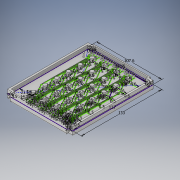
# Autodesk Inventor part: 24WellOneLayerFluidics5x4V2
Saved by Autodesk Inventor 2018 (Build 220112000, 112)
## iProperties
Created: 2019-12-20
Part Number: 24WellOneLayerFluidics5x4V2
Material: Generic
Document SubType Name: Modeling
Designer: Sergio
Density: 1 g/cm^3
Appearance: Default
Author: Sergio
Autodesk Inventor part; units mm, degrees
(part 1 of 4)
ref_plane "YZ Plane" through (0, 0, 0) normal (1, 0, 0) x (0, 1, 0)
ref_plane "XZ Plane" through (0, 0, 0) normal (0, 1, 0) x (-1, 0, 0)
ref_plane "XY Plane" through (0, 0, 0) normal (0, 0, 1) x (1, 0, 0)
sketch "Sketch2" plane through (0, 0, 0) normal (0, 1, 0) x (-1, 0, 0)
  line L0 (-50.8, 63.5) -> (-50.8, -63.5) construction
  line L1 (-50.8, -63.5) -> (50.8, -63.5) construction
  line L2 (50.8, -63.5) -> (50.8, 63.5) construction
  line L3 (50.8, 63.5) -> (-50.8, 63.5) construction
  line L4 (-50.8, 63.5) -> (50.8, -63.5) construction
  line L5 (-50.8, -63.5) -> (50.8, 63.5) construction
  line L6 (-53.8, 66.5) -> (-53.8, -66.5) construction
  line L7 (-53.8, -66.5) -> (53.8, -66.5) construction
  line L8 (53.8, -66.5) -> (53.8, 66.5) construction
  line L9 (53.8, 66.5) -> (-53.8, 66.5) construction
  line L10 (-53.8, 66.5) -> (53.8, -66.5) construction
  line L11 (-53.8, -66.5) -> (53.8, 66.5) construction
  line L12 (53.8, 66.5) -> (46.8, 66.5) construction
  line L13 (50.8, 63.5) -> (44.8, 63.5) construction
  line L14 (44.8, 63.5) -> (44.8, 67) construction
  line L15 (46.8, 66.5) -> (46.8, 69) construction
  line L16 (-53.8, 66.5) -> (-46.8, 66.5) construction
  line L17 (-50.8, 63.5) -> (-44.8, 63.5) construction
  line L18 (-46.8, 66.5) -> (-46.8, 69) construction
  line L19 (-44.8, 63.5) -> (-44.8, 67) construction
  line L20 (-53.8, -66.5) -> (-46.8, -66.5) construction
  line L21 (-50.8, -63.5) -> (-44.8, -63.5) construction
  line L22 (-46.8, -66.5) -> (-46.8, -69) construction
  line L23 (-44.8, -63.5) -> (-44.8, -67) construction
  line L24 (53.8, -66.5) -> (46.8, -66.5) construction
  line L25 (50.8, -63.5) -> (44.8, -63.5) construction
  line L26 (46.8, -66.5) -> (46.8, -69) construction
  line L27 (44.8, -63.5) -> (44.8, -67) construction
  line L28 (46.8, 69) -> (-46.8, 69) construction
  line L29 (-44.8, 67) -> (44.8, 67) construction
  line L30 (44.8, -67) -> (-44.8, -67) construction
  line L31 (-46.8, -69) -> (46.8, -69) construction
  point P0 (0, 0)
  dimension "d21" = 127
  dimension "d22" = 101.6
  dimension "d23" = 133
  dimension "d24" = 107.6
  dimension "d25" = 7
  dimension "d26" = 6
  dimension "d27" = 3.5
  dimension "d28" = 2.5
  dimension "d29" = 7
  dimension "d30" = 6
  dimension "d31" = 2.5
  dimension "d32" = 3.5
  dimension "d33" = 7
  dimension "d34" = 6
  dimension "d35" = 2.5
  dimension "d36" = 3.5
  dimension "d37" = 7
  dimension "d38" = 6
  dimension "d39" = 2.5
  dimension "d40" = 3.5
  constraints: 64 end point, 9 vertical, 8 point on line, 4 midpoint, 4 parallel, 3 perpendicular
  measures "d21" distance of L0.start L0.end
  measures "d22" distance of L1.end L0.end
  measures "d23" distance of L6.start L6.end
  measures "d24" distance of L7.end L6.end
  measures "d25" distance of L8.end L12.end
  measures "d26" distance of L2.end L13.end
  measures "d27" distance of L13.end L14.end
  measures "d28" distance of L12.end L15.end
  measures "d29" distance of L6.start L16.end
  measures "d30" distance of L0.start L17.end
  measures "d31" distance of L16.end L18.end
  measures "d32" distance of L17.end L19.end
  measures "d33" distance of L6.end L20.end
  measures "d34" distance of L0.end L21.end
  measures "d35" distance of L20.end L22.end
  measures "d36" distance of L21.end L23.end
  measures "d37" distance of L7.end L24.end
  measures "d38" distance of L1.end L25.end
  measures "d39" distance of L24.end L26.end
  measures "d40" distance of L25.end L27.end
sketch "Sketch3" plane through (0, 0, 0) normal (0, 1, 0) x (-1, 0, 0)
  line L0 (50.8, 63.5) -> (-50.8, 63.5) construction
  line L1 (-50.8, -63.5) -> (50.8, -63.5) construction
  line L2 (50.8, -63.5) -> (50.8, 63.5) construction
  line L3 (-53.8, 66.5) -> (-53.8, -66.5) construction
  line L4 (53.8, -66.5) -> (53.8, 66.5) construction
  line L5 (53.8, 66.5) -> (-53.8, 66.5) construction
  line L6 (-44.8, 67) -> (44.8, 67) construction
  line L7 (46.8, 69) -> (-46.8, 69) construction
  line L8 (-46.8, -69) -> (46.8, -69) construction
  line L9 (44.8, -67) -> (-44.8, -67) construction
  line L10 (46.8, 69) -> (-46.8, 69)
  line L11 (46.8, -69) -> (-46.8, -69)
  line L12 (46.8, 66.5) -> (46.8, 69) construction
  line L13 (44.8, 63.5) -> (44.8, 67) construction
  line L14 (50.8, 63.5) -> (44.8, 63.5) construction
  line L15 (53.8, 66.5) -> (46.8, 66.5) construction
  line L16 (46.8, 69) -> (46.8, 66.5)
  line L17 (46.8, 66.5) -> (53.8, 66.5)
  line L18 (53.8, 66.5) -> (53.8, -66.5)
  line L19 (53.8, -66.5) -> (46.8, -66.5)
  line L20 (46.8, -66.5) -> (46.8, -69)
  line L21 (-46.8, -69) -> (-46.8, -66.5)
  line L22 (-46.8, -66.5) -> (-53.8, -66.5)
  line L23 (-53.8, 66.5) -> (-53.8, -66.5)
  line L24 (-46.8, 69) -> (-46.8, 66.5)
  line L25 (-53.8, 66.5) -> (-46.8, 66.5)
  line L26 (-44.8, 67) -> (-44.8, 63.5)
  line L27 (-44.8, 63.5) -> (-50.8, 63.5)
  line L28 (-50.8, 63.5) -> (-50.8, -63.5) construction
  line L29 (-44.8, -63.5) -> (-44.8, -67) construction
  line L30 (-44.8, -63.5) -> (-44.8, -67)
  line L31 (-44.8, -63.5) -> (-50.8, -63.5)
  line L32 (-50.8, -63.5) -> (-50.8, 63.5)
  line L33 (-44.8, 67) -> (44.8, 67)
  line L34 (44.8, 67) -> (44.8, 63.5)
  line L35 (44.8, 63.5) -> (50.8, 63.5)
  line L36 (50.8, 63.5) -> (50.8, -63.5)
  line L37 (50.8, -63.5) -> (44.8, -63.5)
  line L38 (44.8, -63.5) -> (44.8, -67)
  line L39 (44.8, -67) -> (-44.8, -67)
  line L40 (44.8, 63.5) -> (-44.8, 63.5)
  line L41 (44.8, -63.5) -> (-44.8, -63.5)
  line L42 (-44.8, -63.5) -> (44.8, -63.5)
  line L43 (44.8, -63.5) -> (44.8, -64.25)
  line L44 (44.8, -64.25) -> (-44.8, -64.25)
  line L45 (-44.8, -64.25) -> (-44.8, -63.5)
  point P0 (0, 0)
  dimension "d547" = 89.6
  dimension "d548" = 0.75
  constraints: 60 end point, 11 perpendicular, 9 collinear, 7 point on line, 5 parallel, 2 horizontal, 1 vertical
  measures "d547" distance of L43.end L44.end
  measures "d548" distance of L42.end L43.end
extrude "Extrusion1" add sketch "Sketch3" along normal blind 6 and the other way blind 8
extrude "Extrusion2" add sketch "Sketch3" against normal blind 8 contours L33 L34 L40 L26 | L40 L35 L36 L37 L41 L31 L32 L27 | L41 L38 L44 L30 | L44 L38 L39 L30
sketch "Sketch5" plane through (0, 0, 0) normal (0, 1, 0) x (1, 0, 0)
  line L0 (-50.8, 63.5) -> (-44.8, 63.5) construction
  line L1 (-50.8, 63.5) -> (-41.305, 63.5) construction
  line L2 (-50.8, 60.019) -> (-50.8, 63.5) construction
  line L3 (-50.8, -63.5) -> (-50.8, 63.5) construction
  line L4 (-50.8, -63.5) -> (-29.25, -63.5) construction
  line L5 (-29.25, -63.5) -> (-29.25, -48.75) construction
  line L6 (-29.25, -48.75) -> (-50.8, -48.75) construction
  line L7 (-50.8, -48.75) -> (-50.8, -63.5) construction
  circle A0 centre (-29.25, -48.75) radius 2.8 construction
  line L8 (-29.25, -48.75) -> (-29.25, -29.25) construction
  circle A1 centre (-29.25, -29.25) radius 2.8 construction
  line L9 (-29.25, -29.25) -> (-29.25, -9.75) construction
  line L10 (-29.25, -9.75) -> (-29.25, 9.75) construction
  line L11 (-29.25, 9.75) -> (-29.25, 29.25) construction
  line L12 (-29.25, 29.25) -> (-29.25, 48.75) construction
  circle A2 centre (-29.25, -9.75) radius 2.8 construction
  circle A3 centre (-29.25, 9.75) radius 2.8 construction
  circle A4 centre (-29.25, 29.25) radius 2.8 construction
  circle A5 centre (-29.25, 48.75) radius 2.8 construction
  line L13 (-29.25, 48.75) -> (-9.75, 48.75) construction
  line L14 (-9.75, 48.75) -> (9.75, 48.75) construction
  line L15 (9.75, 48.75) -> (29.25, 48.75) construction
  circle A6 centre (-9.75, 48.75) radius 2.8 construction
  circle A7 centre (9.75, 48.75) radius 2.8 construction
  circle A8 centre (29.25, 48.75) radius 2.8 construction
  circle A9 centre (-9.75, -48.75) radius 2.8 construction
  circle A10 centre (-9.75, -29.25) radius 2.8 construction
  circle A11 centre (-9.75, -9.75) radius 2.8 construction
  circle A12 centre (-9.75, 9.75) radius 2.8 construction
  circle A13 centre (-9.75, 29.25) radius 2.8 construction
  circle A14 centre (9.75, -48.75) radius 2.8 construction
  circle A15 centre (9.75, -29.25) radius 2.8 construction
  circle A16 centre (9.75, -9.75) radius 2.8 construction
  circle A17 centre (9.75, 9.75) radius 2.8 construction
  circle A18 centre (9.75, 29.25) radius 2.8 construction
  circle A19 centre (29.25, -48.75) radius 2.8 construction
  circle A20 centre (29.25, -29.25) radius 2.8 construction
  circle A21 centre (29.25, -9.75) radius 2.8 construction
  circle A22 centre (29.25, 9.75) radius 2.8 construction
  circle A23 centre (29.25, 29.25) radius 2.8 construction
  circle A24 centre (29.25, 29.25) radius 2.8 construction
  circle A25 centre (29.25, 48.75) radius 2.8 construction
  circle A26 centre (29.25, -29.25) radius 2.8 construction
  circle A27 centre (29.25, -48.75) radius 2.8 construction
  line L16 (26.45, -48.75) -> (25.391, -48.75) construction
  line L17 (-29.2495, -4.9541) -> (-29.2495, -4.4541) construction
  point P0 (0, 0)
  dimension "d49" = 21.55
  dimension "d50" = 14.75
  dimension "d51" = 5.6
  dimension "d52" = 19.5
  dimension "d53" = 5.6
  dimension "d54" = 19.5
  dimension "d55" = 19.5
  dimension "d56" = 19.5
  dimension "d57" = 19.5
  dimension "d58" = 5.6
  dimension "d59" = 5.6
  dimension "d60" = 5.6
  dimension "d61" = 5.6
  dimension "d62" = 19.5
  dimension "d63" = 19.5
  dimension "d64" = 19.5
  dimension "d65" = 5.6
  dimension "d66" = 5.6
  dimension "d67" = 5.6
  dimension "d68" = 5.6
  dimension "d69" = 5.6
  dimension "d70" = 5.6
  dimension "d71" = 5.6
  dimension "d72" = 5.6
  dimension "d73" = 5.6
  dimension "d74" = 5.6
  dimension "d75" = 5.6
  dimension "d76" = 5.6
  dimension "d77" = 5.6
  dimension "d78" = 5.6
  dimension "d79" = 5.6
  dimension "d80" = 5.6
  dimension "d81" = 5.6
  dimension "d82" = 5.6
  dimension "d88" = 1.059
  constraints: 32 end point, 27 centre point, 9 coincident, 5 point on line, 3 horizontal, 2 parallel, 2 vertical, 1 horizontal alignment, 1 perpendicular, 2 other
  measures "d49" distance of L6.end L5.end
  measures "d50" distance of L5.end L4.end
  measures "d51" diameter of A0
  measures "d52" distance of L8.start L8.end
  measures "d53" diameter of A1
  measures "d54" distance of L9.start L9.end
  measures "d55" distance of L9.end L10.end
  measures "d56" distance of L10.end L11.end
  measures "d57" distance of L11.end L12.end
  measures "d58" diameter of A2
  measures "d59" diameter of A3
  measures "d60" diameter of A4
  measures "d61" diameter of A5
  measures "d62" distance of L13.start L13.end
  measures "d63" distance of L13.end L14.end
  measures "d64" distance of L14.end L15.end
  measures "d65" diameter of A6
  measures "d66" diameter of A7
  measures "d67" diameter of A8
  measures "d68" diameter of A9
  measures "d69" diameter of A10
  measures "d70" diameter of A11
  measures "d71" diameter of A12
  measures "d72" diameter of A13
  measures "d73" diameter of A14
  measures "d74" diameter of A15
  measures "d75" diameter of A16
  measures "d76" diameter of A17
  measures "d77" diameter of A18
  measures "d78" diameter of A19
  measures "d79" diameter of A20
  measures "d80" diameter of A21
  measures "d81" diameter of A22
  measures "d82" diameter of A23
  measures "d88" distance of L16.start L16.end
sketch "Sketch6" plane through (0, 0, 0) normal (0, 1, 0) x (1, 0, 0)
  circle A0 centre (35.0419, -55.5191) radius 0.75 construction
  line L0 (35.0419, -55.5191) -> (35.0419, -60.0514) construction
  circle A1 centre (37.3055, -60.0191) radius 0.75 construction
  circle A2 centre (33.3055, -60.0191) radius 0.75 construction
  line L1 (33.3055, -60.0191) -> (37.3055, -60.0191) construction
  circle A3 centre (29.25, 29.25) radius 2.8 construction
  circle A4 centre (29.25, 48.75) radius 2.8 construction
  circle A5 centre (29.25, -29.25) radius 2.8 construction
  circle A6 centre (29.25, -48.75) radius 2.8 construction
  circle A7 centre (29.3055, -60.0191) radius 0.75 construction
  line L2 (34.4097, -49.3098) -> (34.4156, -25.002) construction
  line L3 (35.7822, -49.2776) -> (35.7822, -7.8641) construction
  line L4 (37.0912, 9.3686) -> (37.0912, -49.2776) construction
  line L5 (38.4002, 26.6014) -> (38.4002, -49.2776) construction
  line L6 (26.45, -48.75) -> (25.391, -48.75) construction
  line L7 (33.3055, -60.0191) -> (37.3055, -60.0191) construction
  line L8 (35.0419, -55.5191) -> (39.0419, -55.5191) construction
  line L9 (37.3055, -60.0191) -> (41.3055, -60.0191) construction
  circle A8 centre (41.3055, -60.0191) radius 0.75 construction
  line L10 (29.25, -35.55) -> (33.1642, -42.2012) construction
  line L11 (34.4097, -49.3098) -> (35.0419, -50.4326) construction
  line L12 (35.0419, -55.5191) -> (35.0419, -50.4326) construction
  line L13 (29.25, -16.05) -> (34.4156, -25.002) construction
  line L14 (37.3055, -60.0191) -> (37.3055, -51.916) construction
  line L15 (29.25, 3.45) -> (35.7822, -7.8641) construction
  line L16 (29.25, 22.95) -> (37.0912, 9.3686) construction
  line L17 (29.25, 42.45) -> (38.4002, 26.6014) construction
  line L18 (39.0419, -55.5191) -> (39.0419, -52.6564) construction
  line L19 (39.0419, -52.6564) -> (37.0912, -49.2776) construction
  line L20 (41.3055, -60.0191) -> (41.3055, -54.3097) construction
  line L21 (38.4002, -49.2776) -> (41.3055, -54.3097) construction
  line L22 (35.7822, -49.2776) -> (37.3055, -51.916) construction
  line L23 (33.3055, -60.0191) -> (33.3055, -49.5223) construction
  line L24 (33.1642, -42.2012) -> (33.1642, -49.2776) construction
  line L25 (33.1642, -49.2776) -> (33.3055, -49.5223) construction
  line L26 (29.25, -53.55) -> (29.25, -48.75) construction
  line L27 (29.25, -53.55) -> (29.25, -54.05) construction
  line L28 (29.25, -34.05) -> (29.25, -29.25) construction
  line L29 (29.25, -34.05) -> (29.25, -34.55) construction
  line L30 (29.25, 4.95) -> (29.25, 9.75) construction
  line L31 (29.25, 4.95) -> (29.25, 4.45) construction
  line L32 (29.25, 24.45) -> (29.25, 29.25) construction
  line L33 (29.25, 24.45) -> (29.25, 23.95) construction
  line L34 (29.25, 43.95) -> (29.25, 48.75) construction
  line L35 (29.25, 43.95) -> (29.25, 43.45) construction
  line L36 (29.25, -14.55) -> (29.25, -15.05) construction
  line L37 (29.25, -14.55) -> (29.25, -9.75) construction
  line L38 (29.3055, -60.0191) -> (29.3055, -54.0496) construction
  line L39 (29.25, 43.45) -> (29.25, 42.45) construction
  line L40 (29.25, 23.95) -> (29.25, 22.95) construction
  line L41 (29.25, 4.45) -> (29.25, 3.45) construction
  line L42 (29.25, -34.55) -> (29.25, -35.55) construction
  line L43 (29.25, -15.05) -> (29.25, -16.05) construction
  circle A9 centre (39.0419, -55.5191) radius 0.75 construction
  line L44 (29.25, -34.05) -> (29.25, -34.85) construction
  line L45 (29.25, -34.85) -> (30.65, -34.85) construction
  line L46 (30.65, -34.85) -> (30.65, -34.05) construction
  line L47 (30.65, -34.05) -> (29.25, -34.05) construction
  line L48 (29.25, -34.05) -> (29.25, -34.85) construction
  line L49 (29.25, -34.85) -> (27.85, -34.85) construction
  line L50 (27.85, -34.85) -> (27.85, -34.05) construction
  line L51 (27.85, -34.05) -> (29.25, -34.05) construction
  line L52 (29.25, -15.35) -> (30.65, -15.35) construction
  line L53 (30.65, -15.35) -> (30.65, -14.55) construction
  line L54 (30.65, -14.55) -> (29.25, -14.55) construction
  line L55 (29.25, -15.35) -> (27.85, -15.35) construction
  line L56 (27.85, -15.35) -> (27.85, -14.55) construction
  line L57 (27.85, -14.55) -> (29.25, -14.55) construction
  line L58 (29.25, 4.15) -> (30.65, 4.15) construction
  line L59 (30.65, 4.15) -> (30.65, 4.95) construction
  line L60 (30.65, 4.95) -> (29.25, 4.95) construction
  line L61 (29.25, 4.15) -> (27.85, 4.15) construction
  line L62 (27.85, 4.15) -> (27.85, 4.95) construction
  line L63 (27.85, 4.95) -> (29.25, 4.95) construction
  line L64 (29.25, 23.65) -> (30.65, 23.65) construction
  line L65 (30.65, 23.65) -> (30.65, 24.45) construction
  line L66 (30.65, 24.45) -> (29.25, 24.45) construction
  line L67 (29.25, 23.65) -> (27.85, 23.65) construction
  line L68 (27.85, 23.65) -> (27.85, 24.45) construction
  line L69 (27.85, 24.45) -> (29.25, 24.45) construction
  line L70 (29.25, 43.15) -> (30.65, 43.15) construction
  line L71 (30.65, 43.15) -> (30.65, 43.95) construction
  line L72 (30.65, 43.95) -> (29.25, 43.95) construction
  line L73 (29.25, 43.15) -> (27.85, 43.15) construction
  line L74 (27.85, 43.15) -> (27.85, 43.95) construction
  line L75 (27.85, 43.95) -> (29.25, 43.95) construction
  line L76 (30.65, -53.55) -> (29.25, -53.55) construction
  line L77 (30.65, -54.35) -> (30.65, -53.55) construction
  line L78 (29.25, -54.35) -> (30.65, -54.35) construction
  line L79 (27.85, -53.55) -> (29.25, -53.55) construction
  line L80 (27.85, -54.35) -> (27.85, -53.55) construction
  line L81 (29.25, -54.35) -> (27.85, -54.35) construction
  point P0 (0, 0)
  dimension "d106" = 1.5
  dimension "d107" = 1.5
  dimension "d108" = 1.5
  dimension "d109" = 1.5
  dimension "d110" = 4
  dimension "d111" = 1.059
  dimension "d112" = 4
  dimension "d113" = 4.5
  dimension "d114" = 4
  dimension "d115" = 1.5
  dimension "d116" = 4
  dimension "d117" = 4.8
  dimension "d118" = 4.8
  dimension "d119" = 4.8
  dimension "d120" = 4.8
  dimension "d121" = 4.8
  dimension "d122" = 4.8
  dimension "d123" = 1
  dimension "d124" = 1
  dimension "d125" = 1
  dimension "d126" = 1
  dimension "d127" = 1
  dimension "d128" = 1.5
  dimension "d129" = 0.8
  dimension "d130" = 1.4
  dimension "d131" = 1.4
  dimension "d132" = 0.8
  dimension "d133" = 1.4
  dimension "d134" = 1.4
  dimension "d135" = 0.8
  dimension "d136" = 1.4
  dimension "d137" = 1.4
  dimension "d138" = 0.8
  dimension "d139" = 1.4
  dimension "d140" = 1.4
  dimension "d141" = 0.8
  dimension "d142" = 1.4
  dimension "d143" = 1.4
  dimension "d144" = 0.8
  dimension "d145" = 1.4
  dimension "d146" = 1.4
  constraints: 164 end point, 15 vertical, 14 parallel, 9 centre point, 8 point on line, 3 horizontal, 3 perpendicular, 2 coincident, 1 horizontal alignment, 2 other
  measures "d106" diameter of A0
  measures "d107" diameter of A1
  measures "d108" diameter of A2
  measures "d109" diameter of A7
  measures "d110" distance of L38.start L1.start
  measures "d111" distance of L6.start L6.end
  measures "d112" distance of L8.start L8.end
  measures "d113" distance between parallel lines of L1 L8
  measures "d114" distance of L9.start L9.end
  measures "d115" diameter of A8
  measures "d116" distance of L1.start L1.end
  measures "d117" distance of L26.start L26.end
  measures "d118" distance of L29.start L28.end
  measures "d119" distance of L31.start L30.end
  measures "d120" distance of L33.start L32.end
  measures "d121" distance of L35.start L34.end
  measures "d122" distance of L36.start L37.end
  measures "d123" distance of L35.end L39.end
  measures "d124" distance of L33.end L40.end
  measures "d125" distance of L31.end L41.end
  measures "d126" distance of L29.end L42.end
  measures "d127" distance of L43.start L43.end
  measures "d128" diameter of A9
  measures "d129" distance of L29.start L44.end
  measures "d130" distance of L45.end L44.end
  measures "d131" distance of L44.end L49.end
  measures "d132" distance of L54.end L52.start
  measures "d133" distance of L53.start L52.start
  measures "d134" distance of L52.start L56.start
  measures "d135" distance of L60.end L58.start
  measures "d136" distance of L59.start L58.start
  measures "d137" distance of L58.start L62.start
  measures "d138" distance of L66.end L64.start
  measures "d139" distance of L65.start L64.start
  measures "d140" distance of L64.start L68.start
  measures "d141" distance of L72.end L70.start
  measures "d142" distance of L71.start L70.start
  measures "d143" distance of L70.start L74.start
  measures "d144" distance of L79.end L81.start
  measures "d145" distance of L77.start L81.start
  measures "d146" distance of L81.start L80.start
sketch "Sketch7" plane through (0, 0, 0) normal (0, 1, 0) x (1, 0, 0)
  line L0 (34.4097, -49.3098) -> (34.4156, -25.002) construction
  line L1 (38.4002, -49.2776) -> (41.3055, -54.3097) construction
  circle A0 centre (29.3055, -60.0191) radius 0.75 construction
  circle A1 centre (33.3055, -60.0191) radius 0.75 construction
  circle A2 centre (35.0419, -55.5191) radius 0.75 construction
  circle A3 centre (37.3055, -60.0191) radius 0.75 construction
  circle A4 centre (39.0419, -55.5191) radius 0.75 construction
  circle A5 centre (41.3055, -60.0191) radius 0.75 construction
  line L2 (41.3055, -60.0191) -> (41.3055, -54.3097) construction
  line L3 (38.1502, -49.2107) -> (38.1502, 26.4004)
  line L4 (38.6502, 26.5344) -> (38.6502, -49.0767)
  line L5 (40.9885, -54.2607) -> (38.2172, -49.4607)
  line L6 (38.7172, -49.3267) -> (41.4885, -54.1267)
  line L7 (41.089, -54.4347) -> (38.6167, -49.1526) construction
  line L8 (38.1837, -49.4026) -> (41.522, -54.1847) construction
  line L9 (41.0555, -60.0187) -> (41.0555, -54.5107)
  line L10 (41.5555, -54.3767) -> (41.5555, -60.0187)
  line L11 (41.5555, -60.0187) -> (41.0555, -60.0187)
  line L12 (41.0555, -60.0187) -> (41.5555, -54.3101) construction
  line L13 (41.0555, -54.3101) -> (41.5555, -60.0187) construction
  line L14 (38.7919, -55.5191) -> (38.7919, -52.8573)
  line L15 (39.2919, -52.7233) -> (39.2919, -55.5191)
  line L16 (39.2919, -55.5191) -> (38.7919, -55.5191)
  line L17 (38.7919, -55.5191) -> (39.2919, -52.6564) construction
  line L18 (38.7919, -52.6564) -> (39.2919, -55.5191) construction
  line L19 (38.7249, -52.6073) -> (36.9082, -49.4607)
  line L20 (37.4082, -49.3267) -> (39.2249, -52.4733)
  line L21 (38.8254, -52.7814) -> (37.3077, -49.1526) construction
  line L22 (36.8747, -49.4026) -> (39.2584, -52.5314) construction
  line L23 (35.5992, -49.4607) -> (36.9885, -51.867)
  line L24 (37.4885, -51.733) -> (36.0992, -49.3267)
  line L25 (35.5657, -49.4026) -> (37.522, -51.791) construction
  line L26 (37.089, -52.041) -> (35.9987, -49.1526) construction
  line L27 (37.0555, -52.117) -> (37.0555, -60.0191)
  line L28 (37.0555, -60.0191) -> (37.5555, -60.0191)
  line L29 (37.5555, -60.0191) -> (37.5555, -51.983)
  line L30 (37.0555, -51.916) -> (37.5555, -60.0191) construction
  line L31 (37.0555, -60.0191) -> (37.5555, -51.916) construction
  line L32 (36.8412, 9.1677) -> (36.8412, -49.2107)
  line L33 (37.3412, -49.0767) -> (37.3412, 9.3016)
  line L34 (36.8412, 9.3686) -> (37.3412, -49.2776) construction
  line L35 (36.8412, -49.2776) -> (37.3412, 9.3686) construction
  line L36 (35.5322, -49.2107) -> (35.5322, -8.0651)
  line L37 (36.0322, -7.9311) -> (36.0322, -49.0767)
  line L38 (35.5322, -49.2776) -> (36.0322, -7.8641) construction
  line L39 (35.5322, -7.8641) -> (36.0322, -49.2776) construction
  line L40 (34.7919, -55.5191) -> (34.7919, -50.6197)
  line L41 (35.2919, -50.4857) -> (35.2919, -55.5191)
  line L42 (35.2919, -55.5191) -> (34.7919, -55.5191)
  line L43 (34.7919, -55.5191) -> (35.2919, -50.4326) construction
  line L44 (34.7919, -50.4326) -> (35.2919, -55.5191) construction
  line L45 (34.7249, -50.3697) -> (34.2296, -49.5118)
  line L46 (34.7296, -49.3778) -> (35.2249, -50.2357)
  line L47 (34.8314, -50.5541) -> (34.6202, -49.1883) construction
  line L48 (34.1872, -49.4383) -> (35.2644, -50.3041) construction
  line L49 (33.5555, -60.0191) -> (33.5555, -49.5893)
  line L50 (33.0555, -49.7233) -> (33.0555, -60.0191)
  line L51 (33.0555, -60.0191) -> (33.5555, -60.0191)
  line L52 (33.5555, -60.0191) -> (33.0555, -49.5223) construction
  line L53 (33.5555, -49.5223) -> (33.0555, -60.0191) construction
  line L54 (32.9812, -49.4607) -> (32.9885, -49.4733)
  line L55 (33.4885, -49.3393) -> (33.4812, -49.3267)
  circle A6 centre (41.3055, -60.0191) radius 0.75
  circle A7 centre (37.3055, -60.0191) radius 0.75
  circle A8 centre (39.0419, -55.5191) radius 0.75
  circle A9 centre (35.0419, -55.5191) radius 0.75
  circle A10 centre (33.3055, -60.0191) radius 0.75
  circle A11 centre (29.3055, -60.0191) radius 0.75
  line L56 (32.9142, -42.4055) -> (32.9142, -49.2107)
  line L57 (33.4142, -49.0767) -> (33.4142, -42.2693)
  line L58 (32.9142, -42.2012) -> (33.4142, -49.2776) construction
  line L59 (32.9142, -49.2776) -> (33.4142, -42.2012) construction
  line L60 (34.1626, -25.1978) -> (34.1626, -49.2618)
  line L61 (34.6626, -49.1278) -> (34.6626, -25.0639)
  line L62 (34.1626, -25.002) -> (34.6626, -49.3098) construction
  line L63 (34.1626, -49.3098) -> (34.6626, -25.002) construction
  arc A12 (33.5555, -49.5893) -> (33.4885, -49.3393) centre (33.0555, -49.5893) ccw
  arc A13 (33.0555, -49.7233) -> (32.9885, -49.4733) centre (32.5555, -49.7233) ccw
  arc A14 (32.9142, -49.2107) -> (32.9812, -49.4607) centre (33.4142, -49.2107) ccw
  arc A15 (33.4142, -49.0767) -> (33.4812, -49.3267) centre (33.9142, -49.0767) ccw
  arc A16 (34.6626, -49.1278) -> (34.7296, -49.3778) centre (35.1626, -49.1278) ccw
  arc A17 (34.1626, -49.2618) -> (34.2296, -49.5118) centre (34.6626, -49.2618) ccw
  arc A18 (36.0322, -49.0767) -> (36.0992, -49.3267) centre (36.5322, -49.0767) ccw
  arc A19 (35.5322, -49.2107) -> (35.5992, -49.4607) centre (36.0322, -49.2107) ccw
  arc A20 (36.8412, -49.2107) -> (36.9082, -49.4607) centre (37.3412, -49.2107) ccw
  arc A21 (37.3412, -49.0767) -> (37.4082, -49.3267) centre (37.8412, -49.0767) ccw
  arc A22 (38.6502, -49.0767) -> (38.7172, -49.3267) centre (39.1502, -49.0767) ccw
  arc A23 (38.1502, -49.2107) -> (38.2172, -49.4607) centre (38.6502, -49.2107) ccw
  arc A24 (35.2919, -50.4857) -> (35.2249, -50.2357) centre (34.7919, -50.4857) ccw
  arc A25 (34.7919, -50.6197) -> (34.7249, -50.3697) centre (34.2919, -50.6197) ccw
  arc A26 (37.0555, -52.117) -> (36.9885, -51.867) centre (36.5555, -52.117) ccw
  arc A27 (37.5555, -51.983) -> (37.4885, -51.733) centre (37.0555, -51.983) ccw
  arc A28 (39.2919, -52.7233) -> (39.2249, -52.4733) centre (38.7919, -52.7233) ccw
  arc A29 (38.7919, -52.8573) -> (38.7249, -52.6073) centre (38.2919, -52.8573) ccw
  arc A30 (41.0555, -54.5107) -> (40.9885, -54.2607) centre (40.5555, -54.5107) ccw
  arc A31 (41.5555, -54.3767) -> (41.4885, -54.1267) centre (41.0555, -54.3767) ccw
  line L64 (29.25, 42.45) -> (38.4002, 26.6014) construction
  line L65 (29.067, 42.267) -> (38.0832, 26.6504)
  line L66 (38.1837, 26.4764) -> (38.6167, 26.7264)
  line L67 (38.5832, 26.7844) -> (29.567, 42.401)
  line L68 (29.0335, 42.325) -> (38.6167, 26.7264) construction
  line L69 (38.1837, 26.4764) -> (29.4665, 42.575) construction
  arc A32 (38.6502, 26.5344) -> (38.5832, 26.7844) centre (38.1502, 26.5344) ccw
  arc A33 (38.1502, 26.4004) -> (38.0832, 26.6504) centre (37.6502, 26.4004) ccw
  line L70 (30.65, 43.15) -> (30.65, 43.95) construction
  line L71 (30.65, 43.95) -> (29.25, 43.95) construction
  line L72 (29.25, 43.15) -> (30.65, 43.15) construction
  line L73 (30.65, 43.95) -> (30.65, 43.15)
  line L74 (27.85, 43.15) -> (27.85, 43.95)
  line L75 (27.85, 43.95) -> (30.65, 43.95)
  line L76 (29, 43.15) -> (29, 42.517)
  line L77 (29.5, 42.651) -> (29.5, 43.15)
  line L78 (29, 43.15) -> (29.5, 42.45) construction
  line L79 (29, 42.45) -> (29.5, 43.15) construction
  arc A34 (29.5, 42.651) -> (29.567, 42.401) centre (30, 42.651) ccw
  arc A35 (29, 42.517) -> (29.067, 42.267) centre (29.5, 42.517) ccw
  line L80 (29.25, 22.95) -> (37.0912, 9.3686) construction
  line L81 (29.067, 22.767) -> (36.7742, 9.4177)
  line L82 (36.8747, 9.2436) -> (37.3077, 9.4936)
  line L83 (37.2742, 9.5516) -> (29.567, 22.901)
  line L84 (29.4665, 23.075) -> (29.0335, 22.825)
  line L85 (29.0335, 22.825) -> (37.3077, 9.4936) construction
  line L86 (36.8747, 9.2436) -> (29.4665, 23.075) construction
  arc A36 (37.3412, 9.3016) -> (37.2742, 9.5516) centre (36.8412, 9.3016) ccw
  arc A37 (36.8412, 9.1677) -> (36.7742, 9.4177) centre (36.3412, 9.1677) ccw
  line L87 (29.25, 3.45) -> (35.7822, -7.8641) construction
  line L88 (29.25, -35.55) -> (33.1642, -42.2012) construction
  line L89 (29.25, -16.05) -> (34.4156, -25.002) construction
  line L90 (29.0669, -16.2329) -> (34.0957, -24.9479)
  line L91 (34.5957, -24.814) -> (29.5669, -16.099)
  line L92 (29.4665, -15.9251) -> (29.0335, -16.1749)
  line L93 (29.0335, -16.1749) -> (34.6321, -24.8771) construction
  line L94 (34.199, -25.127) -> (29.4665, -15.9251) construction
  line L95 (29.0691, -35.7355) -> (32.8451, -42.1519)
  line L96 (33.3451, -42.0157) -> (29.5691, -35.5993)
  line L97 (29.0345, -35.6768) -> (33.3797, -42.0744) construction
  line L98 (32.9487, -42.328) -> (29.4655, -35.4232) construction
  line L99 (29.067, 3.267) -> (35.4652, -7.8151)
  line L100 (35.9652, -7.6811) -> (29.567, 3.401)
  line L101 (29.4665, 3.575) -> (29.0335, 3.325)
  line L102 (29.0335, 3.325) -> (35.9987, -7.7391) construction
  line L103 (35.5657, -7.9891) -> (29.4665, 3.575) construction
  arc A38 (36.0322, -7.9311) -> (35.9652, -7.6811) centre (35.5322, -7.9311) ccw
  arc A39 (35.5322, -8.0651) -> (35.4652, -7.8151) centre (35.0322, -8.0651) ccw
  arc A40 (34.6626, -25.0639) -> (34.5957, -24.814) centre (34.1626, -25.0639) ccw
  arc A41 (34.1626, -25.1978) -> (34.0957, -24.9479) centre (33.6626, -25.1978) ccw
  arc A42 (33.4142, -42.2693) -> (33.3451, -42.0157) centre (32.9142, -42.2693) ccw
  arc A43 (32.9142, -42.4055) -> (32.8451, -42.1519) centre (32.4142, -42.4055) ccw
  line L104 (30.65, 23.65) -> (30.65, 24.45) construction
  line L105 (30.65, 4.15) -> (30.65, 4.95) construction
  line L106 (30.65, 4.95) -> (29.25, 4.95) construction
  line L107 (30.65, -15.35) -> (30.65, -14.55) construction
  line L108 (30.65, -14.55) -> (29.25, -14.55) construction
  line L109 (27.85, -15.35) -> (27.85, -14.55) construction
  line L110 (29.25, -15.35) -> (27.85, -15.35) construction
  line L111 (30.65, -34.85) -> (30.65, -34.05) construction
  line L112 (30.65, -34.05) -> (29.25, -34.05) construction
  line L113 (27.85, -34.85) -> (27.85, -34.05) construction
  line L114 (29.25, -34.85) -> (27.85, -34.85) construction
  line L115 (29.25, -15.35) -> (29.25, -16.05)
  line L116 (29.25, 4.15) -> (30.65, 4.15) construction
  line L117 (29, 23.65) -> (29, 23.017)
  line L118 (29, 22.95) -> (29.5, 22.95)
  line L119 (29.5, 23.151) -> (29.5, 23.65)
  line L120 (29, 23.65) -> (29.5, 22.95) construction
  line L121 (29, 22.95) -> (29.5, 23.65) construction
  line L122 (29, 4.15) -> (29, 3.517)
  line L123 (29, 3.45) -> (29.5, 3.45)
  line L124 (29.5, 3.651) -> (29.5, 4.15)
  line L125 (29, -15.35) -> (29, -15.983)
  line L126 (29, -16.05) -> (29.5, -16.05)
  line L127 (29.5, -15.8491) -> (29.5, -15.35)
  line L128 (29, -15.35) -> (29.5, -16.05) construction
  line L129 (29, -16.05) -> (29.5, -15.35) construction
  line L130 (29, -34.85) -> (29, -35.4819)
  line L131 (29.5, -35.3457) -> (29.5, -34.85)
  line L132 (29, -34.85) -> (29.5, -35.55) construction
  line L133 (29, -35.55) -> (29.5, -34.85) construction
  line L134 (30.65, 24.45) -> (27.85, 24.45)
  line L135 (27.85, 24.45) -> (27.85, 23.65)
  line L136 (30.65, 23.65) -> (30.65, 24.45)
  line L137 (29.25, 4.15) -> (27.85, 4.15) construction
  line L138 (30.65, 4.95) -> (27.85, 4.95)
  line L139 (27.85, 4.95) -> (27.85, 4.15)
  line L140 (30.65, 4.15) -> (30.65, 4.95)
  line L141 (30.65, -14.55) -> (27.85, -14.55)
  line L142 (27.85, -14.55) -> (27.85, -15.35)
  line L143 (30.65, -15.35) -> (30.65, -14.55)
  line L144 (30.65, -34.05) -> (27.85, -34.05)
  line L145 (27.85, -34.05) -> (27.85, -34.85)
  line L146 (30.65, -34.85) -> (30.65, -34.05)
  arc A44 (29.5, 23.151) -> (29.567, 22.901) centre (30, 23.151) ccw
  arc A45 (29, 23.017) -> (29.067, 22.767) centre (29.5, 23.017) ccw
  arc A46 (29.5, 3.651) -> (29.567, 3.401) centre (30, 3.651) ccw
  arc A47 (29, 3.517) -> (29.067, 3.267) centre (29.5, 3.517) ccw
  arc A48 (29.5, -15.8491) -> (29.5669, -16.099) centre (30, -15.8491) ccw
  arc A49 (29, -15.983) -> (29.0669, -16.2329) centre (29.5, -15.983) ccw
  arc A50 (29, -35.4819) -> (29.0691, -35.7355) centre (29.5, -35.4819) ccw
  arc A51 (29.5, -35.3457) -> (29.5691, -35.5993) centre (30, -35.3457) ccw
  line L147 (27.85, -34.85) -> (29, -34.85)
  line L148 (29.5, -34.85) -> (30.65, -34.85)
  line L149 (30.65, -54.35) -> (30.65, -53.55) construction
  line L150 (30.65, -53.55) -> (29.25, -53.55) construction
  line L151 (27.85, -54.35) -> (27.85, -53.55) construction
  line L152 (30.65, -53.55) -> (27.85, -53.55)
  line L153 (27.85, -53.55) -> (27.85, -54.35)
  line L154 (30.65, -54.35) -> (30.65, -53.55)
  line L155 (29.0705, -60.0191) -> (29.0705, -54.35)
  line L156 (29.5555, -54.35) -> (29.5555, -60.0191)
  line L157 (29.5555, -60.0191) -> (29.0705, -60.0191)
  line L158 (29.0705, -60.0191) -> (29.5168, -54.35) construction
  line L159 (29.0705, -54.2285) -> (29.5555, -60.0191) construction
  line L160 (27.85, -54.35) -> (29.0705, -54.35)
  line L161 (29.5555, -54.35) -> (30.65, -54.35)
  line L162 (30.65, 43.15) -> (29.5, 43.15)
  line L163 (29, 43.15) -> (27.85, 43.15)
  line L164 (27.85, 23.65) -> (29, 23.65)
  line L165 (29.5, 23.65) -> (30.65, 23.65)
  line L166 (27.85, 4.15) -> (29, 4.15)
  line L167 (29.5, 4.15) -> (30.65, 4.15)
  line L168 (27.85, -15.35) -> (29, -15.35)
  line L169 (29.5, -15.35) -> (30.65, -15.35)
  line L170 (29.25, 43.95) -> (29.25, 48.75) construction
  line L171 (29.25, 48.75) -> (29.25, 43.95)
  circle A52 centre (29.25, -48.75) radius 2.8 construction
  line L172 (29.5, 43.15) -> (29, 43.15)
  line L173 (29.5, 23.65) -> (29, 23.65)
  line L174 (29.5, 4.15) -> (29, 4.15)
  line L175 (29.5, -15.35) -> (29, -15.35)
  line L176 (29.5, -34.85) -> (29, -34.85)
  line L177 (29.0705, -54.35) -> (29.5555, -54.35)
  line L178 (27.85, 54.35) -> (27.85, 53.55)
  line L179 (28.9445, 54.35) -> (27.85, 54.35)
  line L180 (27.85, 53.55) -> (30.65, 53.55)
  line L181 (30.65, 54.35) -> (29.4295, 54.35)
  line L182 (30.65, 53.55) -> (30.65, 54.35)
  line L183 (28.9445, 54.35) -> (28.9445, 60.0191)
  line L184 (28.9445, 60.0191) -> (29.4295, 60.0191)
  line L185 (29.4295, 60.0191) -> (29.4295, 54.35)
  line L186 (29.4295, 60.0191) -> (28.9832, 54.35) construction
  line L187 (29.4295, 54.2285) -> (28.9445, 60.0191) construction
  line L188 (29.4295, 54.35) -> (28.9445, 54.35)
  circle A53 centre (29.1945, 60.0191) radius 0.75
  line L189 (16.9445, 60.0187) -> (17.4445, 60.0187)
  circle A54 centre (17.1945, 60.0191) radius 0.75
  line L190 (21.4445, 60.0191) -> (20.9445, 60.0191)
  circle A55 centre (21.1945, 60.0191) radius 0.75
  line L191 (25.4445, 60.0191) -> (24.9445, 60.0191)
  circle A56 centre (25.1945, 60.0191) radius 0.75
  arc A57 (19.7081, 52.8573) -> (19.7751, 52.6073) centre (20.2081, 52.8573) ccw
  arc A58 (19.2081, 52.7233) -> (19.2751, 52.4733) centre (19.7081, 52.7233) ccw
  line L192 (19.7081, 55.5191) -> (19.7081, 52.8573)
  line L193 (19.7081, 55.5191) -> (19.2081, 52.6564) construction
  line L194 (19.7081, 52.6564) -> (19.2081, 55.5191) construction
  line L195 (19.2081, 55.5191) -> (19.7081, 55.5191)
  circle A59 centre (19.4581, 55.5191) radius 0.75
  line L196 (21.4445, 60.0191) -> (20.9445, 51.916) construction
  line L197 (21.4445, 51.916) -> (20.9445, 60.0191) construction
  line L198 (21.4445, 52.117) -> (21.4445, 60.0191)
  line L199 (20.9445, 60.0191) -> (20.9445, 51.983)
  line L200 (17.4445, 60.0187) -> (17.4445, 54.5107)
  line L201 (17.4445, 60.0187) -> (16.9445, 54.3101) construction
  line L202 (17.4445, 54.3101) -> (16.9445, 60.0187) construction
  line L203 (16.9445, 54.3767) -> (16.9445, 60.0187)
  line L204 (19.2081, 52.7233) -> (19.2081, 55.5191)
  line L205 (23.2081, 55.5191) -> (23.7081, 55.5191)
  circle A60 centre (23.4581, 55.5191) radius 0.75
  line L206 (25.4445, 49.7233) -> (25.4445, 60.0191)
  line L207 (24.9445, 60.0191) -> (25.4445, 49.5223) construction
  line L208 (24.9445, 49.5223) -> (25.4445, 60.0191) construction
  line L209 (24.9445, 60.0191) -> (24.9445, 49.5893)
  line L210 (23.7081, 55.5191) -> (23.7081, 50.6197)
  line L211 (23.2081, 50.4857) -> (23.2081, 55.5191)
  line L212 (23.7081, 55.5191) -> (23.2081, 50.4326) construction
  line L213 (23.7081, 50.4326) -> (23.2081, 55.5191) construction
  arc A61 (23.2081, 50.4857) -> (23.2751, 50.2357) centre (23.7081, 50.4857) ccw
  arc A62 (23.7081, 50.6197) -> (23.7751, 50.3697) centre (24.2081, 50.6197) ccw
  arc A63 (17.4445, 54.5107) -> (17.5115, 54.2607) centre (17.9445, 54.5107) ccw
  arc A64 (16.9445, 54.3767) -> (17.0115, 54.1267) centre (17.4445, 54.3767) ccw
  arc A65 (19.8498, 49.0767) -> (19.7828, 49.3267) centre (19.3498, 49.0767) ccw
  line L214 (17.411, 54.4347) -> (19.8833, 49.1526) construction
  line L215 (17.5115, 54.2607) -> (20.2828, 49.4607)
  line L216 (19.7828, 49.3267) -> (17.0115, 54.1267)
  line L217 (20.3163, 49.4026) -> (16.978, 54.1847) construction
  arc A66 (21.6588, 49.2107) -> (21.5918, 49.4607) centre (21.1588, 49.2107) ccw
  arc A67 (21.1588, 49.0767) -> (21.0918, 49.3267) centre (20.6588, 49.0767) ccw
  arc A68 (20.3498, 49.2107) -> (20.2828, 49.4607) centre (19.8498, 49.2107) ccw
  line L218 (22.9008, 49.4607) -> (21.5115, 51.867)
  line L219 (22.9343, 49.4026) -> (20.978, 51.791) construction
  line L220 (21.411, 52.041) -> (22.5013, 49.1526) construction
  line L221 (21.0115, 51.733) -> (22.4008, 49.3267)
  line L222 (19.6746, 52.7814) -> (21.1923, 49.1526) construction
  line L223 (19.7751, 52.6073) -> (21.5918, 49.4607)
  line L224 (21.0918, 49.3267) -> (19.2751, 52.4733)
  line L225 (21.6253, 49.4026) -> (19.2416, 52.5314) construction
  arc A69 (21.4445, 52.117) -> (21.5115, 51.867) centre (21.9445, 52.117) ccw
  arc A70 (20.9445, 51.983) -> (21.0115, 51.733) centre (21.4445, 51.983) ccw
  line L226 (23.7704, 49.3778) -> (23.2751, 50.2357)
  line L227 (23.6686, 50.5541) -> (23.8798, 49.1883) construction
  arc A71 (23.8374, 49.1278) -> (23.7704, 49.3778) centre (23.3374, 49.1278) ccw
  arc A72 (25.0858, 49.0767) -> (25.0188, 49.3267) centre (24.5858, 49.0767) ccw
  line L228 (25.0115, 49.3393) -> (25.0188, 49.3267)
  arc A73 (25.5858, 49.2107) -> (25.5188, 49.4607) centre (25.0858, 49.2107) ccw
  arc A74 (24.9445, 49.5893) -> (25.0115, 49.3393) centre (25.4445, 49.5893) ccw
  arc A75 (25.4445, 49.7233) -> (25.5115, 49.4733) centre (25.9445, 49.7233) ccw
  arc A76 (24.3374, 49.2618) -> (24.2704, 49.5118) centre (23.8374, 49.2618) ccw
  line L229 (23.7751, 50.3697) -> (24.2704, 49.5118)
  line L230 (24.3128, 49.4383) -> (23.2356, 50.3041) construction
  line L231 (25.5188, 49.4607) -> (25.5115, 49.4733)
  arc A77 (22.4678, 49.0767) -> (22.4008, 49.3267) centre (21.9678, 49.0767) ccw
  arc A78 (22.9678, 49.2107) -> (22.9008, 49.4607) centre (22.4678, 49.2107) ccw
  arc A79 (25.5858, 42.4055) -> (25.6549, 42.1519) centre (26.0858, 42.4055) ccw
  line L232 (25.5858, 42.4055) -> (25.5858, 49.2107)
  line L233 (25.0858, 49.0767) -> (25.0858, 42.2693)
  line L234 (25.5858, 49.2776) -> (25.0858, 42.2012) construction
  line L235 (25.5858, 42.2012) -> (25.0858, 49.2776) construction
  arc A80 (25.0858, 42.2693) -> (25.1549, 42.0157) centre (25.5858, 42.2693) ccw
  line L236 (25.5513, 42.328) -> (29.0345, 35.4232) construction
  line L237 (25.1549, 42.0157) -> (28.9309, 35.5993)
  line L238 (29.4655, 35.6768) -> (25.1203, 42.0744) construction
  line L239 (29.4309, 35.7355) -> (25.6549, 42.1519)
  arc A81 (29, 35.3457) -> (28.9309, 35.5993) centre (28.5, 35.3457) ccw
  arc A82 (29.5, 35.4819) -> (29.4309, 35.7355) centre (29, 35.4819) ccw
  line L240 (29, 35.3457) -> (29, 34.85)
  line L241 (29, 34.85) -> (27.85, 34.85)
  line L242 (27.85, 34.85) -> (27.85, 34.05)
  line L243 (29.5, 34.85) -> (29, 35.55) construction
  line L244 (29.5, 35.55) -> (29, 34.85) construction
  line L245 (29.5, 34.85) -> (29.5, 35.4819)
  line L246 (27.85, 34.05) -> (30.65, 34.05)
  line L247 (29, 34.85) -> (29.5, 34.85)
  line L248 (30.65, 34.85) -> (29.5, 34.85)
  line L249 (30.65, 34.05) -> (30.65, 34.85)
  line L250 (27.85, 14.55) -> (30.65, 14.55)
  line L251 (27.85, 15.35) -> (27.85, 14.55)
  line L252 (29, 15.35) -> (27.85, 15.35)
  line L253 (29, 15.35) -> (29.5, 15.35)
  line L254 (30.65, 14.55) -> (30.65, 15.35)
  line L255 (30.65, 15.35) -> (29.5, 15.35)
  line L256 (29, 15.8491) -> (29, 15.35)
  line L257 (29.5, 15.35) -> (29.5, 15.983)
  line L258 (29.25, 15.35) -> (29.25, 16.05)
  line L259 (29.5, 15.35) -> (29, 16.05) construction
  line L260 (29.5, 16.05) -> (29, 15.35) construction
  line L261 (29.5, 16.05) -> (29, 16.05)
  arc A83 (29, 15.8491) -> (28.9331, 16.099) centre (28.5, 15.8491) ccw
  line L262 (29.0335, 15.9251) -> (29.4665, 16.1749)
  arc A84 (29.5, 15.983) -> (29.4331, 16.2329) centre (29, 15.983) ccw
  arc A85 (29.5, -3.517) -> (29.433, -3.267) centre (29, -3.517) ccw
  line L263 (29.0335, -3.575) -> (29.4665, -3.325)
  line L264 (29.433, -3.267) -> (23.0348, 7.8151)
  line L265 (29.4665, -3.325) -> (22.5013, 7.7391) construction
  line L266 (22.5348, 7.6811) -> (28.933, -3.401)
  line L267 (22.9343, 7.9891) -> (29.0335, -3.575) construction
  arc A86 (22.9678, 8.0651) -> (23.0348, 7.8151) centre (23.4678, 8.0651) ccw
  arc A87 (22.4678, 7.9311) -> (22.5348, 7.6811) centre (22.9678, 7.9311) ccw
  arc A88 (29, -3.651) -> (28.933, -3.401) centre (28.5, -3.651) ccw
  line L268 (29.5, -3.45) -> (29, -3.45)
  line L269 (29, -3.651) -> (29, -4.15)
  line L270 (29.5, -4.15) -> (29.5, -3.517)
  line L271 (29, -4.15) -> (27.85, -4.15)
  line L272 (29, -4.15) -> (29.5, -4.15)
  line L273 (30.65, -4.15) -> (29.5, -4.15)
  line L274 (27.85, -4.15) -> (27.85, -4.95)
  line L275 (27.85, -4.95) -> (30.65, -4.95)
  line L276 (30.65, -4.95) -> (30.65, -4.15)
  arc A89 (21.6588, -9.1677) -> (21.7258, -9.4177) centre (22.1588, -9.1677) ccw
  arc A90 (21.1588, -9.3016) -> (21.2258, -9.5516) centre (21.6588, -9.3016) ccw
  line L277 (19.8498, -26.5344) -> (19.8498, 49.0767)
  line L278 (20.3498, 49.2107) -> (20.3498, -26.4004)
  line L279 (21.1588, 49.0767) -> (21.1588, -9.3016)
  line L280 (21.6588, 49.2776) -> (21.1588, -9.3686) construction
  line L281 (21.6588, -9.3686) -> (21.1588, 49.2776) construction
  line L282 (21.6588, -9.1677) -> (21.6588, 49.2107)
  line L283 (22.4678, 7.9311) -> (22.4678, 49.0767)
  line L284 (22.9678, 7.8641) -> (22.4678, 49.2776) construction
  line L285 (22.9678, 49.2776) -> (22.4678, 7.8641) construction
  line L286 (22.9678, 49.2107) -> (22.9678, 8.0651)
  line L287 (23.8374, 49.1278) -> (23.8374, 25.0639)
  line L288 (24.3374, 25.1978) -> (24.3374, 49.2618)
  line L289 (24.3374, 49.3098) -> (23.8374, 25.002) construction
  line L290 (24.3374, 25.002) -> (23.8374, 49.3098) construction
  line L291 (29.0335, -23.075) -> (29.4665, -22.825)
  line L292 (21.2258, -9.5516) -> (28.933, -22.901)
  line L293 (21.6253, -9.2436) -> (29.0335, -23.075) construction
  line L294 (29.4665, -22.825) -> (21.1923, -9.4936) construction
  line L295 (21.6253, -9.2436) -> (21.1923, -9.4936)
  line L296 (29.433, -22.767) -> (21.7258, -9.4177)
  line L297 (29, -23.65) -> (29.5, -23.65)
  line L298 (29, -23.151) -> (29, -23.65)
  line L299 (29.5, -23.65) -> (29.5, -23.017)
  line L300 (29.5, -23.65) -> (29, -22.95) construction
  line L301 (29.5, -22.95) -> (29, -22.95)
  line L302 (29.5, -22.95) -> (29, -23.65) construction
  arc A91 (29, -23.151) -> (28.933, -22.901) centre (28.5, -23.151) ccw
  line L303 (27.85, -24.45) -> (30.65, -24.45)
  arc A92 (29.5, -23.017) -> (29.433, -22.767) centre (29, -23.017) ccw
  line L304 (30.65, -23.65) -> (29.5, -23.65)
  line L305 (30.65, -24.45) -> (30.65, -23.65)
  arc A93 (20.3498, -26.4004) -> (20.4168, -26.6504) centre (20.8498, -26.4004) ccw
  line L306 (29, -23.65) -> (27.85, -23.65)
  line L307 (27.85, -23.65) -> (27.85, -24.45)
  line L308 (29.433, -42.267) -> (20.4168, -26.6504)
  line L309 (29.4665, -42.325) -> (19.8833, -26.7264) construction
  line L310 (20.3163, -26.4764) -> (29.0335, -42.575) construction
  line L311 (19.9168, -26.7844) -> (28.933, -42.401)
  arc A94 (19.8498, -26.5344) -> (19.9168, -26.7844) centre (20.3498, -26.5344) ccw
  line L312 (20.3163, -26.4764) -> (19.8833, -26.7264)
  line L313 (29.25, -48.75) -> (29.25, -43.95)
  line L314 (30.65, -43.95) -> (27.85, -43.95)
  line L315 (30.65, -43.15) -> (30.65, -43.95)
  arc A95 (29, -42.651) -> (28.933, -42.401) centre (28.5, -42.651) ccw
  arc A96 (29.5, -42.517) -> (29.433, -42.267) centre (29, -42.517) ccw
  line L316 (29, -42.651) -> (29, -43.15)
  line L317 (27.85, -43.15) -> (29, -43.15)
  line L318 (27.85, -43.95) -> (27.85, -43.15)
  line L319 (29.5, -43.15) -> (29.5, -42.517)
  line L320 (29.5, -42.45) -> (29, -43.15) construction
  line L321 (29, -43.15) -> (29.5, -43.15)
  line L322 (29.5, -43.15) -> (30.65, -43.15)
  line L323 (29.5, -43.15) -> (29, -42.45) construction
  line L324 (29.4331, 16.2329) -> (24.4043, 24.9479)
  line L325 (29.4665, 16.1749) -> (23.8679, 24.8771) construction
  line L326 (24.301, 25.127) -> (29.0335, 15.9251) construction
  line L327 (23.9043, 24.814) -> (28.9331, 16.099)
  arc A97 (24.3374, 25.1978) -> (24.4043, 24.9479) centre (24.8374, 25.1978) ccw
  arc A98 (23.8374, 25.0639) -> (23.9043, 24.814) centre (24.3374, 25.0639) ccw
  circle A99 centre (9.75, -48.75) radius 2.8 construction
  circle A100 centre (-9.75, -48.75) radius 2.8 construction
  circle A101 centre (-29.25, -48.75) radius 2.8 construction
  circle A102 centre (9.75, 48.75) radius 2.8 construction
  circle A103 centre (-9.75, 48.75) radius 2.8 construction
  circle A104 centre (-29.25, 48.75) radius 2.8 construction
  line L328 (8.35, 54.35) -> (8.35, 53.55)
  line L329 (9.4445, 54.35) -> (8.35, 54.35)
  line L330 (8.35, 53.55) -> (11.15, 53.55)
  line L331 (11.15, 54.35) -> (9.9295, 54.35)
  line L332 (11.15, 53.55) -> (11.15, 54.35)
  line L333 (9.4445, 54.35) -> (9.4445, 60.0191)
  line L334 (9.4445, 60.0191) -> (9.9295, 60.0191)
  line L335 (9.9295, 60.0191) -> (9.9295, 54.35)
  line L336 (9.9295, 60.0191) -> (9.4832, 54.35) construction
  line L337 (9.9295, 54.2285) -> (9.4445, 60.0191) construction
  line L338 (9.9295, 54.35) -> (9.4445, 54.35)
  circle A105 centre (9.6945, 60.0191) radius 0.75
  line L339 (-2.5555, 60.0187) -> (-2.0555, 60.0187)
  circle A106 centre (-2.3055, 60.0191) radius 0.75
  line L340 (1.9445, 60.0191) -> (1.4445, 60.0191)
  circle A107 centre (1.6945, 60.0191) radius 0.75
  line L341 (5.9445, 60.0191) -> (5.4445, 60.0191)
  circle A108 centre (5.6945, 60.0191) radius 0.75
  arc A109 (0.2081, 52.8573) -> (0.2751, 52.6073) centre (0.7081, 52.8573) ccw
  arc A110 (-0.2919, 52.7233) -> (-0.2249, 52.4733) centre (0.2081, 52.7233) ccw
  line L342 (0.2081, 55.5191) -> (0.2081, 52.8573)
  line L343 (0.2081, 55.5191) -> (-0.2919, 52.6564) construction
  line L344 (0.2081, 52.6564) -> (-0.2919, 55.5191) construction
  line L345 (-0.2919, 55.5191) -> (0.2081, 55.5191)
  circle A111 centre (-0.0419, 55.5191) radius 0.75
  line L346 (1.9445, 60.0191) -> (1.4445, 51.916) construction
  line L347 (1.9445, 51.916) -> (1.4445, 60.0191) construction
  line L348 (1.9445, 52.117) -> (1.9445, 60.0191)
  line L349 (1.4445, 60.0191) -> (1.4445, 51.983)
  line L350 (-2.0555, 60.0187) -> (-2.0555, 54.5107)
  line L351 (-2.0555, 60.0187) -> (-2.5555, 54.3101) construction
  line L352 (-2.0555, 54.3101) -> (-2.5555, 60.0187) construction
  line L353 (-2.5555, 54.3767) -> (-2.5555, 60.0187)
  line L354 (-0.2919, 52.7233) -> (-0.2919, 55.5191)
  line L355 (3.7081, 55.5191) -> (4.2081, 55.5191)
  circle A112 centre (3.9581, 55.5191) radius 0.75
  line L356 (5.9445, 49.7233) -> (5.9445, 60.0191)
  line L357 (5.4445, 60.0191) -> (5.9445, 49.5223) construction
  line L358 (5.4445, 49.5223) -> (5.9445, 60.0191) construction
  line L359 (5.4445, 60.0191) -> (5.4445, 49.5893)
  line L360 (4.2081, 55.5191) -> (4.2081, 50.6197)
  line L361 (3.7081, 50.4857) -> (3.7081, 55.5191)
  line L362 (4.2081, 55.5191) -> (3.7081, 50.4326) construction
  line L363 (4.2081, 50.4326) -> (3.7081, 55.5191) construction
  arc A113 (3.7081, 50.4857) -> (3.7751, 50.2357) centre (4.2081, 50.4857) ccw
  arc A114 (4.2081, 50.6197) -> (4.2751, 50.3697) centre (4.7081, 50.6197) ccw
  arc A115 (-2.0555, 54.5107) -> (-1.9885, 54.2607) centre (-1.5555, 54.5107) ccw
  arc A116 (-2.5555, 54.3767) -> (-2.4885, 54.1267) centre (-2.0555, 54.3767) ccw
  arc A117 (0.3498, 49.0767) -> (0.2828, 49.3267) centre (-0.1502, 49.0767) ccw
  line L364 (-2.089, 54.4347) -> (0.3833, 49.1526) construction
  line L365 (-1.9885, 54.2607) -> (0.7828, 49.4607)
  line L366 (0.2828, 49.3267) -> (-2.4885, 54.1267)
  line L367 (0.8163, 49.4026) -> (-2.522, 54.1847) construction
  arc A118 (2.1588, 49.2107) -> (2.0918, 49.4607) centre (1.6588, 49.2107) ccw
  arc A119 (1.6588, 49.0767) -> (1.5918, 49.3267) centre (1.1588, 49.0767) ccw
  arc A120 (0.8498, 49.2107) -> (0.7828, 49.4607) centre (0.3498, 49.2107) ccw
  line L368 (3.4008, 49.4607) -> (2.0115, 51.867)
  line L369 (3.4343, 49.4026) -> (1.478, 51.791) construction
  line L370 (1.911, 52.041) -> (3.0013, 49.1526) construction
  line L371 (1.5115, 51.733) -> (2.9008, 49.3267)
  line L372 (0.1746, 52.7814) -> (1.6923, 49.1526) construction
  line L373 (0.2751, 52.6073) -> (2.0918, 49.4607)
  line L374 (1.5918, 49.3267) -> (-0.2249, 52.4733)
  line L375 (2.1253, 49.4026) -> (-0.2584, 52.5314) construction
  arc A121 (1.9445, 52.117) -> (2.0115, 51.867) centre (2.4445, 52.117) ccw
  arc A122 (1.4445, 51.983) -> (1.5115, 51.733) centre (1.9445, 51.983) ccw
  line L376 (4.2704, 49.3778) -> (3.7751, 50.2357)
  line L377 (4.1686, 50.5541) -> (4.3798, 49.1883) construction
  arc A123 (4.3374, 49.1278) -> (4.2704, 49.3778) centre (3.8374, 49.1278) ccw
  arc A124 (5.5858, 49.0767) -> (5.5188, 49.3267) centre (5.0858, 49.0767) ccw